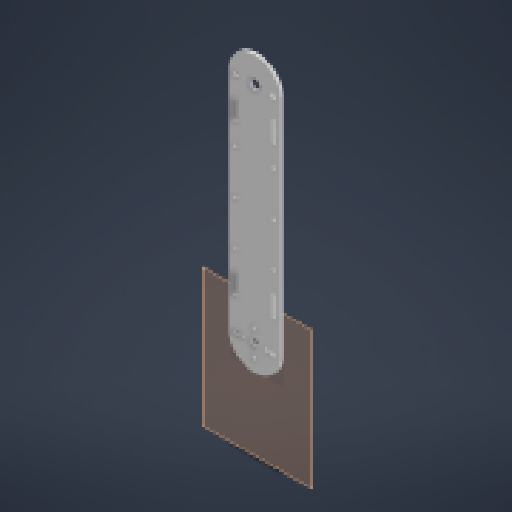
# Autodesk Inventor part: Link2Base
Saved by Autodesk Inventor 2023 (Build 270158000, 158)
## iProperties
Created: 2023-09-09
Part Number: Link2Base
Material: Generic
Document SubType Name: Modeling
Designer: philo
Density: 1 g/cm^3
Appearance: Default
Author: philo
Autodesk Inventor part; units mm, degrees
ref_plane "YZ Plane" through (0, 0, 0) normal (1, 0, 0) x (0, 1, 0)
ref_plane "XZ Plane" through (0, 0, 0) normal (0, 1, 0) x (-1, 0, 0)
ref_plane "XY Plane" through (0, 0, 0) normal (0, 0, 1) x (1, 0, 0)
ref_plane "Work Plane2" through (0.4904, 0, 14) normal (0, 0, 1) x (1, 0, 0)
sketch "Sketch1" plane through (0.4904, 0, 14) normal (0, 0, 1) x (1, 0, 0)
  line L0 (-25, 245.7065) -> (25, 245.7065)
  line L1 (25, 245.7065) -> (25, 5.7065)
  line L2 (25, 5.7065) -> (-25, 5.7065)
  line L3 (-25, 5.7065) -> (-25, 245.7065)
  line L4 (-25, 245.7065) -> (25, 245.7065)
  line L5 (20, 5.7065) -> (-20, 5.7065)
  circle A0 centre (0, 30.7065) radius 3.5 projected
  circle A1 centre (0, 30.7065) radius 25
  circle A2 centre (0, 245.7065) radius 25
  line L6 (-25, 30.7065) -> (-25, 245.7065)
  line L7 (25, 245.7065) -> (25, 30.7065)
  point P0 (-0.4904, 0)
  dimension "d19" = 50
  dimension "d6" = 240
  dimension "d7" = 0
  dimension "d9" = 50
  dimension "d10" = 25
  dimension "d11" = 25
  dimension "d12" = 25
  dimension "d13" = 0
  constraints: 16 end point, 3 parallel, 2 horizontal, 2 point on circle, 2 point on line, 1 centre point, 1 coincident, 1 midpoint, 1 perpendicular, 3 other
  measures "d6" distance between parallel lines of L2 L0
  measures "d7" distance between parallel lines of L0 L4
  measures "d9" diameter of A1
  measures "d10" distance from line of L3 A1.centre
  measures "d11" distance from line of L1 A1.centre
  measures "d12" distance from line of A1.centre L2
  measures "d13" distance between parallel lines of L5 L2
extrude "Extrusion1" add sketch "Sketch1" along normal blind 3 contours A2 L0 | A2 L1 A1 L3 | L0 A2 | A1
sketch "Sketch2" plane through (0.4904, 0, 17) normal (0, 0, 1) x (1, 0, 0)
  arc A0 (25, 245.7065) -> (-25, 245.7065) centre (0, 245.7065) ccw projected
  circle A1 centre (0, 245.7065) radius 5
  point P0 (-0.4904, 0)
  dimension "d16" = 10
  constraints: 1 centre point, 1 coincident
  measures "d16" diameter of A1
extrude "Extrusion2" cut sketch "Sketch2" against normal blind 3
sketch "Sketch3" plane through (0.4904, 0, 17) normal (0, 0, 1) x (1, 0, 0)
  line L0 (-20, 80.7065) -> (-17, 80.7065)
  line L1 (-17, 80.7065) -> (-17, 60.7065)
  line L2 (-17, 60.7065) -> (-20, 60.7065)
  line L3 (-20, 60.7065) -> (-20, 80.7065)
  line L4 (17, 80.7065) -> (20, 80.7065)
  line L5 (20, 80.7065) -> (20, 60.7065)
  line L6 (20, 60.7065) -> (17, 60.7065)
  line L7 (17, 60.7065) -> (17, 80.7065)
  line L8 (25, 30.7065) -> (25, 245.7065) projected
  line L9 (-25, 245.7065) -> (-25, 30.7065) projected
  circle A0 centre (0, 30.7065) radius 3.5 projected
  line L10 (-20, 225.7065) -> (-17, 225.7065)
  line L11 (-17, 225.7065) -> (-17, 205.7065)
  line L12 (-17, 205.7065) -> (-20, 205.7065)
  line L13 (-20, 205.7065) -> (-20, 225.7065)
  line L14 (17, 225.7065) -> (20, 225.7065)
  line L15 (20, 225.7065) -> (20, 205.7065)
  line L16 (20, 205.7065) -> (17, 205.7065)
  line L17 (17, 205.7065) -> (17, 225.7065)
  circle A1 centre (0, 245.7065) radius 5 projected
  circle A2 centre (-18.5, 185.7065) radius 1.5
  circle A3 centre (-18.5, 142.7065) radius 1.5
  circle A4 centre (18.5, 185.7065) radius 1.5
  circle A5 centre (18.5, 142.7065) radius 1.5
  circle A6 centre (18.5, 100.7065) radius 1.5
  circle A7 centre (-18.5, 100.7065) radius 1.5
  point P0 (-0.4904, 0)
  dimension "d20" = 3
  dimension "d21" = 20
  dimension "d22" = 3
  dimension "d23" = 20
  dimension "d24" = 5
  dimension "d25" = 5
  dimension "d26" = 30
  dimension "d27" = 3
  dimension "d28" = 20
  dimension "d29" = 3
  dimension "d30" = 20
  dimension "d31" = 20
  dimension "d32" = 5
  dimension "d33" = 5
  dimension "d34" = 3
  dimension "d35" = 3
  dimension "d36" = 3
  dimension "d37" = 3
  dimension "d38" = 3
  dimension "d39" = 3
  dimension "d40" = 6.5
  dimension "d41" = 6.5
  dimension "d42" = 6.5
  dimension "d43" = 6.5
  dimension "d44" = 6.5
  dimension "d45" = 6.5
  dimension "d46" = 20
  dimension "d47" = 20
  dimension "d48" = 20
  dimension "d49" = 20
  dimension "d50" = 42
  dimension "d51" = 42
  constraints: 32 end point, 8 parallel, 6 centre point, 4 horizontal, 4 perpendicular, 2 point on line
  measures "d20" distance of L1.end L2.end
  measures "d21" distance of L0.end L1.end
  measures "d22" distance of L5.end L6.end
  measures "d23" distance of L4.end L5.end
  measures "d24" distance between parallel lines of L8 L5
  measures "d25" distance between parallel lines of L9 L3
  measures "d26" distance from line of A0.centre L2
  measures "d27" distance of L11.end L12.end
  measures "d28" distance of L10.end L11.end
  measures "d29" distance of L15.end L16.end
  measures "d30" distance of L14.end L15.end
  measures "d31" distance from line of A1.centre L10
  measures "d32" distance between parallel lines of L9 L13
  measures "d33" distance between parallel lines of L8 L15
  measures "d34" diameter of A2
  measures "d35" diameter of A3
  measures "d36" diameter of A4
  measures "d37" diameter of A5
  measures "d38" diameter of A6
  measures "d39" diameter of A7
  measures "d40" distance from line of L8 A4.centre
  measures "d41" distance from line of L8 A5.centre
  measures "d42" distance from line of L8 A6.centre
  measures "d43" distance from line of L9 A7.centre
  measures "d44" distance from line of L9 A3.centre
  measures "d45" distance from line of L9 A2.centre
  measures "d46" distance from line of L12 A2.centre
  measures "d47" distance from line of L16 A4.centre
  measures "d48" distance from line of A6.centre L4
  measures "d49" distance from line of A7.centre L0
  measures "d50" distance of A6.centre A5.centre
  measures "d51" distance of A3.centre A7.centre
extrude "Extrusion3" cut sketch "Sketch3" against normal blind 10 contours L0 L1 L2 L3 | L4 L5 L6 L7 | L10 L11 L12 L13 | L14 L15 L16 L17 | A2 | A3 | A4 | A5 | A6 | A7
sketch "Sketch4" plane through (0.4904, 0, 17) normal (0, 0, 1) x (1, 0, 0)
  arc A0 (20.4946, 25.2317) -> (20.5054, 36.1404) centre (18, 30.6886) ccw projected
  line L0 (20.5054, 36.1404) -> (10.4453, 40.7636) projected
  arc A1 (10.4252, 20.6286) -> (10.4453, 40.7636) centre (0, 30.7065) ccw projected
  line L1 (10.4252, 20.6286) -> (20.4946, 25.2317) projected
  circle A2 centre (18, 30.6886) radius 2.5 projected
  arc A3 (-20.5376, 36.019) -> (-20.4622, 25.1105) centre (-18, 30.582) ccw projected
  line L2 (-20.4622, 25.1105) -> (-11.0226, 20.8627) projected
  arc A4 (-11.1577, 40.3969) -> (-11.0226, 20.8627) centre (0, 30.7065) ccw projected
  line L3 (-11.1577, 40.3969) -> (-20.5376, 36.019) projected
  circle A5 centre (-18, 30.582) radius 2.5 projected
  point P0 (-0.4904, 0)
extrude "Extrusion4" cut sketch "Sketch4" against normal blind 10 contours A2 | A5
sketch "Sketch5" plane through (0.4904, 0, 14) normal (0, 0, -1) x (-1, 0, 0)
  arc A0 (-20.5376, 251.019) -> (-20.4622, 240.1105) centre (-18, 245.582) ccw projected
  line L0 (-20.4622, 240.1105) -> (-11.0226, 235.8627) projected
  arc A1 (-11.1577, 255.3969) -> (-11.0226, 235.8627) centre (0, 245.7065) ccw projected
  line L1 (-11.1577, 255.3969) -> (-20.5376, 251.019) projected
  circle A2 centre (-18, 245.582) radius 2.5 projected
  arc A3 (20.4946, 240.2317) -> (20.5054, 251.1404) centre (18, 245.6886) ccw projected
  line L2 (20.5054, 251.1404) -> (10.4453, 255.7636) projected
  arc A4 (10.4252, 235.6286) -> (10.4453, 255.7636) centre (0, 245.7065) ccw projected
  line L3 (10.4252, 235.6286) -> (20.4946, 240.2317) projected
  circle A5 centre (18, 245.6886) radius 2.5 projected
  point P0 (0.4904, 0)
extrude "Extrusion5" cut sketch "Sketch5" against normal blind 10 contours A2 | A5
sketch "Sketch6" plane through (0.4904, 0, 14) normal (0, 0, -1) x (-1, 0, 0)
  circle A0 centre (0, 42.7065) radius 2 projected
  circle A1 centre (-12, 30.7065) radius 2 projected
  circle A2 centre (0, 18.7065) radius 2 projected
  circle A3 centre (12, 30.7065) radius 2 projected
  point P0 (0.4904, 0)
extrude "Extrusion6" cut sketch "Sketch6" against normal blind 10
body "Solid1"
